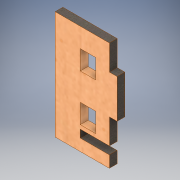
# Autodesk Inventor part: stiffenerDCDC
Saved by Autodesk Inventor 2019 (Build 230136000, 136)
## iProperties
Created: 2021-01-03
Part Number: stiffenerDCDC
Material: Типовые
Document SubType Name: Modeling
Designer: Professional
Density: 1 g/cm^3
Appearance: Вишневое дерево — натуральный — со слабым глянцем
Author: Professional
Autodesk Inventor part; units mm, degrees
ref_plane "YZ Plane" through (0, 0, 0) normal (1, 0, 0) x (0, 1, 0)
ref_plane "XZ Plane" through (0, 0, 0) normal (0, 1, 0) x (-1, 0, 0)
ref_plane "XY Plane" through (0, 0, 0) normal (0, 0, 1) x (1, 0, 0)
sketch "Эскиз1" plane through (0, 0, 0) normal (0, 0, 1) x (1, 0, 0)
  line L0 (0, 0) -> (0, -6)
  line L1 (0, -6) -> (-28, -6)
  line L2 (-28, -6) -> (-28, 50)
  line L3 (-28, 50) -> (0, 50)
  line L4 (0, 50) -> (0, 37)
  line L5 (0, 37) -> (4, 37)
  line L6 (4, 37) -> (4, 17)
  line L7 (4, 17) -> (0, 17)
  line L8 (0, 17) -> (0, 4)
  line L9 (0, 4) -> (-15, 4)
  line L10 (-15, 4) -> (-15, 0)
  line L11 (-15, 0) -> (0, 0)
  line L12 (-7, 6) -> (-15, 6)
  line L13 (-15, 6) -> (-15, 16)
  line L14 (-15, 16) -> (-7, 16)
  line L15 (-7, 16) -> (-7, 6)
  line L16 (-7, 30) -> (-15, 30)
  line L17 (-15, 30) -> (-15, 40)
  line L18 (-15, 40) -> (-7, 40)
  line L19 (-7, 40) -> (-7, 30)
  dimension "d0" = 4
  dimension "d1" = 28
  dimension "d2" = 6
  dimension "d3" = 15
  dimension "d4" = 20
  dimension "d5" = 13
  dimension "d6" = 13
  dimension "d7" = 4
  dimension "d12" = 7
  dimension "d13" = 8
  dimension "d14" = 10
  dimension "d15" = 2
  dimension "d16" = 10
  constraints: 40 end point, 10 perpendicular, 4 parallel, 4 point on line, 3 horizontal, 2 vertical, 1 collinear, 1 vertical alignment
  measures "d0" distance between parallel lines of L9 L11
  measures "d1" distance between parallel lines of L2 L0
  measures "d2" distance between parallel lines of L11 L1
  measures "d3" distance between parallel lines of L0 L10
  measures "d4" distance between parallel lines of L5 L7
  measures "d5" distance between parallel lines of L9 L7
  measures "d6" distance between parallel lines of L3 L5
  measures "d7" distance between parallel lines of L6 L8
  measures "d12" distance between parallel lines of L8 L15
  measures "d13" distance between parallel lines of L15 L13
  measures "d14" distance between parallel lines of L12 L14
  measures "d15" distance between parallel lines of L9 L12
  measures "d16" distance between parallel lines of L3 L18
extrude "Выдавливание1" add sketch "Эскиз1" along normal blind 4
